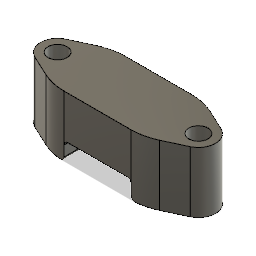
cableClamp (Autodesk Fusion 360 design; units mm, degrees)
Autodesk Fusion 360 part; units mm, degrees
sketch "Sketch1" plane through (0, 0, 0) normal (0, 1, 0) x (1, 0, 0) in component "CableClamp"
  line L0 (0, 0) -> (12, 0)
  line L1 (12, 0) -> (12, -8) construction
  line L2 (12, -8) -> (0, -8)
  line L3 (0, -8) -> (0, 0) construction
  circle A0 centre (15.25, -4) radius 1.25
  circle A1 centre (15.25, -4) radius 2.25
  line L4 (12, -4) -> (13, -4) construction
  line L5 (12, 0) -> (16.2016, -1.9612)
  line L6 (12, -8) -> (16.2016, -6.0388)
  circle A2 centre (-3.25, -4) radius 1.25
  circle A3 centre (-3.25, -4) radius 2.25
  line L7 (0, -4) -> (-1, -4) construction
  line L8 (0, -8) -> (-4.2016, -6.0388)
  line L9 (0, 0) -> (-4.2016, -1.9612)
  dimension "d5" = 12
  dimension "d6" = 8
  dimension "d7" = 2.5
  dimension "d10" = 1
  dimension "d11" = 1
  dimension "d12" = 2.5
  dimension "d13" = 1
  dimension "d14" = 1
  measures "d5" distance of L0.start
  measures "d7" diameter of A0
  measures "d12" diameter of A2
extrude "Extrude1" add sketch "Sketch1" along normal blind 8 in component "CableClamp"
fillet "Fillet1" radius 7.25 4 edges at (0, 4, 0) (12, 4, 0) (12, 4, 8) (0, 4, 8) in component "CableClamp"
sketch "Sketch1 (1)" plane through (0, 0, 8) normal (0, 0, 1) x (1, 0, 0) in component "CableClamp"
  line L0 (1.6087, 8) -> (1.6087, 0)
  line L1 (1.6087, 0) -> (10.3913, 0)
  line L2 (10.3913, 0) -> (10.3913, 8)
  line L3 (10.3913, 8) -> (1.6087, 8)
  line L4 (1.6087, 2.38) -> (10.3913, 2.38)
  dimension "d31" = 2.38
  measures "d31" distance of L1 L4
extrude "Extrude2" cut sketch "Sketch1 (1)" against normal through all contours L0 L1 L2 L4 in component "CableClamp"
fillet "Fillet1'" radius 0.5 4 edges at (1.6087, 2.38, 4) (1.6087, 0, 4) (10.3913, 0, 4) (10.3913, 2.38, 4) in component "CableClamp"
component "CableClamp" placed x (1, 0, 0) y (0, 1, 0) z (0, 0, 1) at (0, 0, 0)
equation "width = 12 mm"
equation "height = 8 mm"
equation "screwHoleDiamerter = 2.5 mm"
equation "screwHoleWallThickness = 1 mm"
equation "d5 = width"
equation "d6 = height"
equation "d7 = screwHoleDiamerter"
equation "d10 = screwHoleWallThickness"
equation "d12 = screwHoleDiamerter"
equation "d13 = screwHoleWallThickness"
equation "thickness = 8 mm"
equation "d16 = thickness"
equation "cableDiameter = 3.4 mm"
equation "clampRatio = 0.7" comment "The closer to 0, the tighter the grip."
equation "d31 = cableDiameter * clampRatio"
